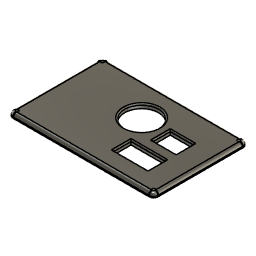
FloppySquare Top (Autodesk Fusion 360 design; units mm, degrees)
part number: 2025-07-31-19-46-25-559
part number: 2025-07-31-19-46-46-452
Autodesk Fusion 360 part; units mm, degrees
sketch "Sketch1" plane through (0, 0, 0) normal (0, 0, 1) x (1, 0, 0) in component "FloppySquare Top (1)"
  line L0 (0, 0) -> (170, 0)
  line L1 (170, 0) -> (170, 110)
  line L2 (170, 110) -> (0, 110)
  line L3 (0, 110) -> (0, 0)
  circle A0 centre (5, 105) radius 1.7
  circle A1 centre (5, 5) radius 1.7
  circle A2 centre (165, 105) radius 1.7
  circle A3 centre (165, 5) radius 1.7
  line L4 (141.5, 75) -> (114.5, 75)
  line L5 (114.5, 75) -> (114.5, 55)
  line L6 (114.5, 55) -> (141.5, 55)
  line L7 (141.5, 55) -> (141.5, 75)
  circle A4 centre (85, 71) radius 20
  line L8 (141.5, 22) -> (101.5, 22)
  line L9 (101.5, 22) -> (101.5, 42)
  line L10 (101.5, 42) -> (141.5, 42)
  line L11 (141.5, 42) -> (141.5, 22)
  dimension "d1" = 170
  dimension "d2" = 110
  dimension "d3" = 3.4
  dimension "d4" = 3.4
  dimension "d5" = 3.4
  dimension "d6" = 3.4
  dimension "d7" = 5
  dimension "d8" = 5
  dimension "d9" = 5
  dimension "d10" = 5
  dimension "d11" = 5
  dimension "d12" = 5
  dimension "d13" = 5
  dimension "d14" = 5
  dimension "d15" = 27
  dimension "d16" = 20
  dimension "d17" = 28.5
  dimension "d18" = 35
  dimension "d19" = 40
  dimension "d20" = 85
  dimension "d21" = 39
  dimension "d22" = 40
  dimension "d23" = 20
  dimension "d24" = 22
  dimension "d25" = 28.5
  constraint horizontal L0
  constraint vertical L1
  constraint horizontal L2
  constraint vertical L3
  constraint coincident L0.start L3.end
  constraint horizontal L4
  constraint vertical L5
  constraint horizontal L6
  constraint vertical L7
  constraint horizontal L8
  constraint vertical L9
  constraint horizontal L10
  constraint vertical L11
  measures "d1" distance of L0.start L0.end
  measures "d2" distance of L0.start L2.end
  measures "d3" diameter of A0
  measures "d4" diameter of A1
  measures "d5" diameter of A2
  measures "d6" diameter of A3
  measures "d7" distance of L0 A3.centre
  measures "d8" distance of L1 A3.centre
  measures "d9" distance of L2 A2.centre
  measures "d10" distance of L1 A2.centre
  measures "d11" distance of L2 A0.centre
  measures "d12" distance of L3 A0.centre
  measures "d13" distance of L0 A1.centre
  measures "d14" distance of L3 A1.centre
  measures "d15" distance of L4.start L4.end
  measures "d16" distance of L4.start L6.end
  measures "d17" distance of L1 L7
  measures "d18" distance of L2 L4
  measures "d19" diameter of A4
  measures "d20" distance of L3 A4.centre
  measures "d21" distance of L2 A4.centre
  measures "d22" distance of L8.start L8.end
  measures "d23" distance of L8.start L10.end
  measures "d24" distance of L0 L8
  measures "d25" distance of L1 L11
extrude "Extrude1" add sketch "Sketch1" along normal blind 5 in component "FloppySquare Top (1)"
fillet "Fillet1" radius 5 4 edges at (0, 110, 2.5) (0, 0, 2.5) (170, 0, 2.5) (170, 110, 2.5) in component "FloppySquare Top (1)"
fillet "Fillet2" radius 3.5 8 edges at (1.4645, 108.5355, 5) (0, 55, 5) (1.4645, 1.4645, 5) (85, 0, 5) (168.5355, 1.4645, 5) (170, 55, 5) (168.5355, 108.5355, 5) (85, 110, 5) in component "FloppySquare Top (1)"
fillet "Fillet3" radius 1.5 9 edges at (141.5, 65, 5) (128, 55, 5) (114.5, 65, 5) (128, 75, 5) (121.5, 42, 5) (141.5, 32, 5) (101.5, 32, 5) (121.5, 22, 5) (66.3535, 78.2323, 5) in component "FloppySquare Top (1)"
component "FloppySquare Top (1)" placed x (1, 0, 0) y (0, 1, 0) z (0, 0, 1) at (0, 0, 0)
